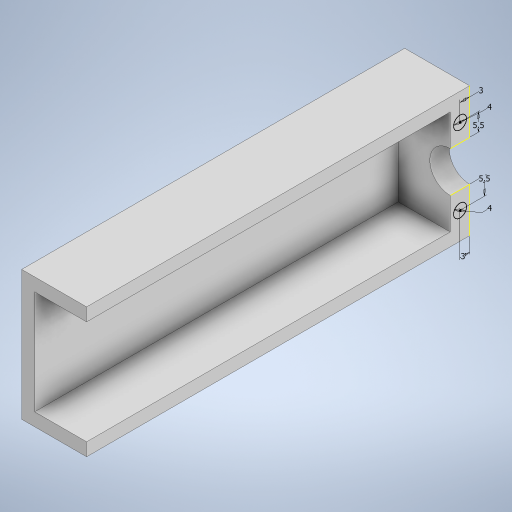
# Autodesk Inventor part: hard_support_m
Saved by Autodesk Inventor 2023 (Build 270158000, 158)
## iProperties
Created: 2024-07-25
Part Number: hard_support_m
Material: 일반
Document SubType Name: Modeling
Designer: ojs08
Density: 1 g/cm^3
Appearance: 기본값
Author: ojs08
Autodesk Inventor part; units mm, degrees
ref_plane "YZ Plane" through (0, 0, 0) normal (1, 0, 0) x (0, 1, 0)
ref_plane "XZ Plane" through (0, 0, 0) normal (0, 1, 0) x (-1, 0, 0)
ref_plane "XY Plane" through (0, 0, 0) normal (0, 0, 1) x (1, 0, 0)
sketch "스케치1" plane through (0, 0, 0) normal (0, 0, 1) x (1, 0, 0)
  line L0 (-20, 40) -> (0, 40)
  line L1 (0, 40) -> (0, 0)
  line L2 (0, 0) -> (-20, 0)
  line L3 (-20, 0) -> (-20, 40)
  circle A0 centre (0, 20) radius 6.25
  line L4 (0, -8) -> (0, 48) projected
  point P0 (0, 13.75)
  point P1 (0, 26.25)
  dimension "d0" = 20
  dimension "d1" = 40
  dimension "d2" = 12.5
  dimension "d3" = 20
  constraints: 8 end point, 2 parallel, 1 centre point, 1 coincident, 1 horizontal, 1 midpoint, 1 perpendicular
  measures "d0" distance of L0.start L0.end
  measures "d1" distance of L2.end L0.start
  measures "d2" diameter of A0
  measures "d3" distance of point (0, 0) A0.centre
extrude "돌출1" add sketch "스케치1" along normal blind 118 contours L0 L1 A0 L2 L3
sketch "스케치2" plane through (0, 0, 118) normal (0, 0, 1) x (1, 0, 0)
  line L0 (0, 40) -> (-20, 40) projected
  line L1 (0, 26.25) -> (0, 40) projected
  arc A0 (0, 26.25) -> (0, 13.75) centre (0, 20) ccw projected
  line L2 (0, 0) -> (0, 13.75) projected
  line L3 (-20, 0) -> (0, 0) projected
  line L4 (0, 36) -> (-16, 36)
  line L5 (-16, 36) -> (-16, 4)
  line L6 (-16, 4) -> (0, 4)
  dimension "d6" = 16
  dimension "d7" = 32
  dimension "d8" = 4
  constraints: 6 end point, 2 perpendicular, 2 point on line, 1 horizontal
  measures "d6" distance of L4.start L4.end
  measures "d7" distance of L4.end L5.end
  measures "d8" distance of L0.start L4.start
extrude "돌출2" cut sketch "스케치2" against normal blind 112
sketch "스케치4" plane through (0, 26.25, 0) normal (1, 0, 0) x (0, 0, -1)
  circle A0 centre (-3, 5.5) radius 2
  circle A1 centre (-3, -18) radius 2
  line L0 (0, -26.25) -> (0, -12.5) projected
  line L1 (0, -12.5) -> (-6, -12.5) projected
  line L2 (0, 0) -> (-6, 0) projected
  line L3 (0, 0) -> (0, 13.75) projected
  dimension "d19" = 4
  dimension "d20" = 4
  dimension "d21" = 3
  dimension "d22" = 5.5
  dimension "d23" = 5.5
  dimension "d24" = 3
  constraints: 2 centre point
  measures "d19" diameter of A0
  measures "d20" diameter of A1
  measures "d21" distance from line of L0 A1.centre
  measures "d22" distance from line of L1 A1.centre
  measures "d23" distance from line of L2 A0.centre
  measures "d24" distance from line of L3 A0.centre
